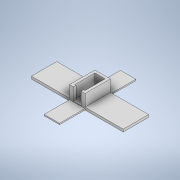
# Autodesk Inventor part: xaxis
Saved by Autodesk Inventor 2021.2 (Build 252289000, 289)
## iProperties
Created: 2021-03-03
Part Number: xaxis
Material: Generic
Document SubType Name: Modeling
Designer: zayda
Density: 1 g/cm^3
Appearance: Default
Author: zayda
Autodesk Inventor part; units mm, degrees
ref_plane "YZ Plane" through (0, 0, 0) normal (1, 0, 0) x (0, 1, 0)
ref_plane "XZ Plane" through (0, 0, 0) normal (0, 1, 0) x (-1, 0, 0)
ref_plane "XY Plane" through (0, 0, 0) normal (0, 0, 1) x (1, 0, 0)
sketch "Sketch1" plane through (0, 0, 0) normal (0, 1, 0) x (-1, 0, 0)
  line L0 (0, 0) -> (-20.5, 0)
  line L1 (-20.5, 0) -> (-20.5, 40.4)
  line L2 (-20.5, 40.4) -> (0, 40.4)
  line L3 (0, 40.4) -> (0, 0)
  line L4 (0, 0) -> (0, -5.08)
  line L5 (0, -5.08) -> (-20.5, -5.08)
  line L6 (-20.5, 0) -> (-20.5, -5.08)
  line L7 (-20.5, -5.08) -> (-25.58, -5.08)
  line L8 (-25.58, -5.08) -> (-25.58, 40.4)
  line L9 (-25.58, 40.4) -> (-25.58, 45.48)
  line L10 (-25.58, 45.48) -> (0, 45.48)
  line L11 (0, 45.48) -> (0, 40.4)
  line L12 (0, -5.08) -> (5.08, -5.08)
  line L13 (5.08, -5.08) -> (5.08, 45.48)
  line L14 (5.08, 45.48) -> (0, 45.48)
  dimension "d0" = 20.5
  dimension "d1" = 40.4
  dimension "d2" = 5.08
  dimension "d3" = 5.08
  dimension "d4" = 5.08
  dimension "d5" = 5.08
  constraints: 30 end point, 7 perpendicular, 4 point on line, 3 parallel, 1 collinear, 1 horizontal, 1 vertical
  measures "d0" distance of L1.end L2.end
  measures "d1" distance of L0.end L1.end
  measures "d2" distance of L0.start L4.end
  measures "d3" distance of L5.end L7.end
  measures "d4" distance of L8.end L9.end
  measures "d5" distance of L4.end L12.end
extrude "Extrusion1" add sketch "Sketch1" along normal blind 25 contours L4 L5 L6 L0 | L3 L11 L14 L13 L12 L4 | L6 L7 L8 L9 L10 L11 L2 L1
sketch "Sketch2" plane through (-5.08, 0, 45.48) normal (0, 0, 1) x (1, 0, 0)
  line L0 (30.66, 0) -> (0, 0) projected
  circle A0 centre (15.33, 0) radius 7.62
  point P0 (5.08, 0)
  point P1 (7.71, 0)
  point P2 (22.95, 0)
  dimension "d8" = 15.24
  constraints: 1 centre point, 1 midpoint
  measures "d8" diameter of A0
extrude "Extrusion2" cut sketch "Sketch2" against normal blind 25 contours L0 A0 picked at (14.7329, 3.7019)
sketch "Sketch3" plane through (0, 0, 0) normal (0, -1, 0) x (1, 0, 0)
  line L0 (25.58, 45.48) -> (25.58, -5.08) projected
  line L1 (25.58, -5.08) -> (-5.08, -5.08) projected
  line L2 (25.58, 45.48) -> (-5.08, 45.48)
  line L3 (-5.08, 45.48) -> (-5.08, -5.08)
  line L4 (-5.08, -5.08) -> (25.58, -5.08)
  line L5 (25.58, -5.08) -> (25.58, 45.48)
  point P0 (0, 0)
  constraints: 8 end point, 2 parallel, 1 horizontal, 1 perpendicular
extrude "Extrusion3" add sketch "Sketch3" along normal blind 3.556
sketch "Sketch4" plane through (25.58, 25, 45.48) normal (1, 0, 0) x (0, 0, -1)
  line L0 (0, -28.556) -> (50.56, -28.556) projected
  line L1 (50.56, -28.556) -> (50.56, 0) projected
  line L2 (0, -28.556) -> (50.56, -28.556)
  line L3 (50.56, -28.556) -> (50.56, -23.4707)
  line L4 (50.56, -23.4707) -> (0, -23.4707)
  line L5 (0, -23.4707) -> (0, -28.556)
  point P0 (45.48, -25)
  constraints: 8 end point, 2 parallel, 1 horizontal, 1 perpendicular, 1 point on line
extrude "Extrusion4" add sketch "Sketch4" along normal blind 76.2
sketch "Sketch5" plane through (-5.08, 25, -5.08) normal (-1, 0, 0) x (0, 0, 1)
  line L0 (50.56, -28.556) -> (0, -28.556) projected
  line L1 (50.56, -23.4707) -> (50.56, 0) projected
  line L2 (0, -28.556) -> (50.56, -28.556)
  line L3 (50.56, -28.556) -> (50.56, -23.4707)
  line L4 (50.56, -23.4707) -> (0, -23.4707)
  line L5 (0, -23.4707) -> (0, -28.556)
  point P0 (5.08, -25)
  constraints: 8 end point, 2 parallel, 1 horizontal, 1 perpendicular
extrude "Extrusion5" add sketch "Sketch5" along normal blind 76.2
sketch "Sketch6" plane through (-5.08, 25, 45.48) normal (0, 0, 1) x (1, 0, 0)
  line L0 (-76.2, -28.556) -> (106.86, -28.556) projected
  line L1 (-0.0136, -28.556) -> (30.66, -28.556)
  line L2 (30.66, -28.556) -> (30.66, -26.016)
  line L3 (30.66, -26.016) -> (-0.0136, -26.016)
  line L4 (-0.0136, -26.016) -> (-0.0136, -28.556)
  point P0 (5.08, -25)
  dimension "d17" = 2.54
  constraints: 8 end point, 2 parallel, 1 horizontal, 1 perpendicular, 1 point on line
  measures "d17" distance of L2.end L1.end
extrude "Extrusion6" add sketch "Sketch6" along normal blind 50.8
sketch "Sketch7" plane through (25.58, 25, -5.08) normal (0, 0, -1) x (-1, 0, 0)
  line L0 (0, -26.016) -> (0, -28.556) projected
  line L1 (30.6736, -26.016) -> (0, -26.016) projected
  line L2 (0, -28.556) -> (30.6736, -28.556)
  line L3 (30.6736, -28.556) -> (30.6736, -26.016)
  line L4 (30.6736, -26.016) -> (0, -26.016)
  line L5 (0, -26.016) -> (0, -28.556)
  point P0 (25.58, -25)
  constraints: 8 end point, 2 parallel, 1 horizontal, 1 perpendicular
extrude "Extrusion7" add sketch "Sketch7" along normal blind 50.8
sketch "Sketch8" plane through (-5.08, 25, 45.48) normal (0, 0, 1) x (1, 0, 0)
  line L0 (7.71, -25) -> (5.08, -25) projected
  line L1 (7.71, -25) -> (7.71, 0)
  line L2 (30.66, 0) -> (0, 0) projected
  line L3 (25.58, -25) -> (22.95, -25) projected
  line L4 (22.95, -25) -> (22.95, 0)
  line L5 (22.95, 0) -> (7.71, 0)
  arc A0 (22.95, -25) -> (7.71, -25) centre (15.33, -25) ccw projected
  line L6 (22.95, -25) -> (7.71, -25) projected
  line L7 (7.71, -25) -> (22.95, -25)
  constraints: 8 end point, 2 vertical, 1 collinear, 1 perpendicular, 1 point on line
extrude "Extrusion8" cut sketch "Sketch8" against normal blind 25.4 contours L1 L2 L4 A0
body "Solid1"
